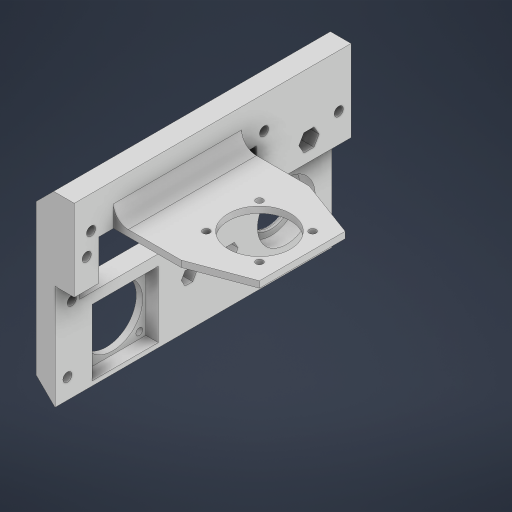
# Autodesk Inventor part: Head_Backplate
Saved by Autodesk Inventor 2024 (Build 280153000, 153)
## iProperties
Created: 2025-09-25
Part Number: Head_Backplate
Material: Generic
Document SubType Name: Modeling
Designer: kevin
Density: 1 g/cm^3
Appearance: Default
Author: kevin
Autodesk Inventor part; units mm, degrees
ref_plane "YZ Plane" through (0, 0, 0) normal (1, 0, 0) x (0, 1, 0)
ref_plane "XZ Plane" through (0, 0, 0) normal (0, 1, 0) x (-1, 0, 0)
sketch "Sketch1" plane through (0, 0, 0) normal (0, 0, 1) x (1, 0, 0)
  line L0 (-40.6109, 70.6994) -> (-33.5378, 59.7448) projected
  line L1 (-33.5378, 59.7448) -> (-15.7647, 71.2203) projected
  line L2 (-15.7647, 71.2203) -> (-15.7647, 87.8486) projected
  line L3 (-15.7647, 87.8486) -> (35.7434, 87.8486) projected
  line L4 (35.7434, 87.8486) -> (-58.3243, 27.112) projected
  line L5 (-58.3243, 27.112) -> (-58.3243, 43.7409) projected
  line L6 (-58.3243, 43.7409) -> (-49.3014, 49.5667) projected
  line L7 (-49.3014, 49.5667) -> (-49.3014, 70.6994) projected
  line L8 (-49.3014, 70.6994) -> (-40.6109, 70.6994) projected
  line L9 (-58.7063, -1.0514) -> (-69.3743, 9.6166) projected
  line L10 (-18.5178, -1.0514) -> (-58.7063, -1.0514) projected
  arc A0 (-21.8066, 1.9486) -> (-18.5178, -1.0514) centre (0, 22.5514) ccw projected
  line L11 (-18.2147, 1.9486) -> (-21.8066, 1.9486) projected
  arc A1 (-18.2147, 1.9486) -> (21.128, 4.9486) centre (0, 22.5514) ccw projected
  line L12 (103.9182, 4.9486) -> (21.128, 4.9486) projected
  line L13 (113.8557, 14.8861) -> (103.9182, 4.9486) projected
  line L14 (113.8557, 93.0111) -> (113.8557, 14.8861) projected
  line L15 (103.9182, 102.9486) -> (113.8557, 93.0111) projected
  line L16 (-46.9118, 102.9486) -> (103.9182, 102.9486) projected
  line L17 (-69.3743, 80.4861) -> (-46.9118, 102.9486) projected
  line L18 (-69.3743, 9.6166) -> (-69.3743, 80.4861) projected
  line L19 (3.2088, 98.8486) -> (52.78, 98.8486) projected
  line L20 (52.78, 98.8486) -> (46.5848, 94.8486) projected
  line L21 (46.5848, 94.8486) -> (5.2088, 94.8486) projected
  line L22 (3.2088, 96.8486) -> (5.2088, 94.8486) projected
  line L23 (3.2088, 96.8486) -> (3.2088, 98.8486) projected
  circle A2 centre (63.0077, 89.467) radius 2.1 projected
  line L24 (67.5987, 76.762) -> (76.5778, 67.7829) projected
  line L25 (76.5778, 67.7829) -> (76.5778, 21.4796) projected
  line L26 (76.5778, 21.4796) -> (68.2692, 13.171) projected
  line L27 (68.2692, 13.171) -> (19.2393, 13.171) projected
  line L28 (19.2393, 13.171) -> (11.6235, 20.7868) projected
  line L29 (11.6235, 20.7868) -> (67.5987, 76.762) projected
  line L30 (-58.0243, 1.9486) -> (-58.0243, 25.3146) projected
  line L31 (-58.0243, -1.0514) -> (-58.0243, 1.9486) projected
  arc A3 (-56.6516, 27.8349) -> (-58.0243, 25.3146) centre (-55.0243, 25.3146) ccw projected
  line L32 (-67.3743, 79.6577) -> (-46.0834, 100.9486)
  line L33 (-46.0834, 100.9486) -> (103.0898, 100.9486)
  line L34 (103.0898, 100.9486) -> (111.8557, 92.1827)
  line L35 (111.8557, 92.1827) -> (111.8557, 15.7145)
  line L36 (111.8557, 15.7145) -> (103.0898, 6.9486)
  line L37 (103.0898, 6.9486) -> (20.1694, 6.9486)
  arc A4 (-17.441, 3.9486) -> (20.1694, 6.9486) centre (0, 22.5514) ccw
  line L38 (-17.441, 3.9486) -> (-26.0372, 3.9486)
  arc A5 (-26.0372, 3.9486) -> (-23.6076, 0.9486) centre (0, 22.5514) ccw
  line L39 (-23.6076, 0.9486) -> (-57.8779, 0.9486)
  line L40 (-57.8779, 0.9486) -> (-67.3743, 10.445) construction
  line L41 (-67.3743, 10.445) -> (-67.3743, 79.6577)
  line L42 (-15.7647, 87.8486) -> (-59.1834, 87.8486)
  line L43 (-49.5014, 70.8994) -> (-49.5014, 49.6757)
  line L44 (-49.5014, 49.6757) -> (-58.5243, 43.8499)
  line L45 (-58.5243, 43.8499) -> (-58.5243, 26.7448)
  line L46 (-58.5243, 26.7448) -> (36.4218, 88.0486)
  line L47 (36.4218, 88.0486) -> (-15.9647, 88.0486)
  line L48 (-15.9647, 88.0486) -> (-15.9647, 71.3293)
  line L49 (-15.9647, 71.3293) -> (-33.4783, 60.0213)
  line L50 (-33.4783, 60.0213) -> (-40.502, 70.8994)
  line L51 (-40.502, 70.8994) -> (-49.5014, 70.8994)
  line L52 (-49.5014, 70.8994) -> (-49.5014, 87.8486)
  line L53 (-58.5243, 26.7448) -> (-58.5243, 1.595)
  line L54 (-67.3743, 9.3192) -> (-58.5243, 0.5765)
  line L55 (-58.5243, 0.5765) -> (-58.5243, 1.595)
  line L56 (-67.3743, 9.3192) -> (-67.3743, 10.445)
  line L57 (-58.5243, 43.8499) -> (-58.5243, 49.6757)
  line L58 (-58.5243, 49.6757) -> (-49.5014, 49.6757)
  point P0 (0, 0)
  dimension "d0" = 2
  dimension "d1" = 0.2
  constraints: 54 end point, 4 point on circle, 3 point on line, 2 centre point, 2 parallel, 2 perpendicular, 1 horizontal, 1 vertical, 19 other
  measures "d0" distance between parallel lines of L18 L41
  measures "d1" distance between parallel lines of L7 L43
ref_plane "Work Plane1" through (-78.2358, -10.3435, 129.6) normal (0, 0, -1) x (0, 1, 0)
extrude "Extrusion1" add sketch "Sketch1" along normal up to surface (129.6 mm away) contours L32 L42 L52 L43 L58 L57 L45 L53 L55 L54 L56 L41
sketch "Sketch2" plane through (-67.3743, 9.3192, 0) normal (-1, 0, 0) x (0, 0, 1)
  circle A0 centre (5.8, 0.6294) radius 2.1 projected
  circle A1 centre (123.8, 0.6294) radius 2.1 projected
  circle A2 centre (123.8, 53.9014) radius 2.1 projected
  circle A3 centre (5.8, 53.9014) radius 2.1 projected
  point P0 (0, -9.3192)
extrude "Extrusion2" cut sketch "Sketch2" against normal blind 25.4
sketch "Sketch4" plane through (-67.3743, 9.3192, 0) normal (-1, 0, 0) x (0, 0, 1)
  arc A0 (125.8035, 0) -> (121.7965, 0) centre (123.8, 0.6294) ccw projected
  line L0 (125.8035, 0) -> (129.6, 0) projected
  line L1 (129.6, 70.3385) -> (129.6, 0) projected
  line L2 (0, 70.3385) -> (129.6, 70.3385) projected
  line L3 (0, 70.3385) -> (0, 0) projected
  line L4 (0, 0) -> (3.7965, 0) projected
  arc A1 (7.8035, 0) -> (3.7965, 0) centre (5.8, 0.6294) ccw projected
  line L5 (7.8035, 0) -> (121.7965, 0) projected
  circle A2 centre (5.8, 53.9014) radius 2.1 projected
  circle A3 centre (123.8, 53.9014) radius 2.1 projected
  circle A4 centre (21.3214, 16.6972) radius 13.5
  point P0 (0, -9.3192)
  dimension "d10" = 27
  constraints: 1 centre point
  measures "d10" diameter of A4
extrude "Extrusion4" cut sketch "Sketch4" against normal up to surface (17.8729 mm away) contours A4
sketch "Sketch5" plane through (-67.3743, 9.3192, 0) normal (-1, 0, 0) x (0, 0, 1)
  circle A0 centre (21.3214, 16.6972) radius 13.5 projected
  circle A1 centre (21.3214, 16.6972) radius 10.325
  point P0 (0, -9.3192)
  dimension "d13" = 20.65
  constraints: 1 centre point, 1 coincident
  measures "d13" diameter of A1
extrude "Extrusion5" add sketch "Sketch5" against normal blind 1.7
fillet "Fillet1" radius 0.6 2 edges at (-67.3743, 26.0164, 10.9964) (-65.6743, 26.0164, 10.9964)
sketch "Sketch7" plane through (-67.3743, 9.3192, 0) normal (-1, 0, 0) x (0, 0, 1)
  circle A0 centre (123.8, 53.9014) radius 2.1 projected
  circle A1 centre (5.8, 53.9014) radius 2.1 projected
  arc A2 (125.8035, 0) -> (121.7965, 0) centre (123.8, 0.6294) ccw projected
  line L0 (125.8035, 0) -> (129.6, 0) projected
  line L1 (129.6, 70.3385) -> (129.6, 0) projected
  line L2 (0, 70.3385) -> (129.6, 70.3385) projected
  line L3 (0, 70.3385) -> (0, 0) projected
  line L4 (0, 0) -> (3.7965, 0) projected
  arc A3 (7.8035, 0) -> (3.7965, 0) centre (5.8, 0.6294) ccw projected
  line L5 (7.8035, 0) -> (121.7965, 0) projected
  circle A4 centre (21.3214, 16.6972) radius 10.925 projected
  circle A5 centre (5.8, 53.9014) radius 3.75
  circle A6 centre (5.8, 0.6294) radius 3.75
  circle A7 centre (123.8, 0.6294) radius 3.75
  circle A8 centre (123.8, 53.9014) radius 3.75
  circle A9 centre (5.8, 0.6294) radius 2.1 projected
  line L6 (2.8, -0.8456) -> (126.8, -0.8456) construction
  circle A10 centre (123.8, 0.6294) radius 2.1 projected
  point P0 (0, -9.3192)
  point P1 (120.1032, 0)
  point P2 (127.4968, 0)
  point P3 (2.1032, 0)
  point P4 (9.4968, 0)
  dimension "d19" = 7.5
  dimension "d20" = 7.5
  dimension "d21" = 7.5
  dimension "d22" = 7.5
  constraints: 4 centre point, 4 coincident
  measures "d19" diameter of A5
  measures "d20" diameter of A6
  measures "d21" diameter of A7
  measures "d22" diameter of A8
extrude "Extrusion7" add sketch "Sketch7" against normal up to surface contours L0 A7 L5 A10 | A6 L4 A9 L5 surface through (-67.3743, 9.3192, 0) normal (-0.7027793, -0.7114079, 0)
sketch "Sketch9" plane through (-67.3743, 9.3192, 0) normal (-1, 0, 0) x (0, 0, 1)
  circle A0 centre (123.8, 53.9014) radius 3.75 projected
  circle A1 centre (5.8, 53.9014) radius 2.1 projected
  circle A2 centre (5.8, 53.9014) radius 3.75
  point P0 (0, -9.3192)
  dimension "d40" = 7.5
  dimension "d41" = 7.5
  constraints: 1 centre point, 1 coincident
  measures "d40" diameter of A2
  measures "d41" diameter of A0
extrude "Extrusion9" cut sketch "Sketch9" against normal blind 4
sketch "Sketch10" plane through (-67.3743, 9.3192, 0) normal (-1, 0, 0) x (0, 0, 1)
  line L0 (50.2647, 59.1822) -> (50.2647, 34.7978) projected
  arc A0 (54.9397, 63.8572) -> (50.2647, 59.1822) centre (54.9397, 59.1822) ccw projected
  line L1 (107.5897, 63.8572) -> (54.9397, 63.8572) projected
  arc A1 (112.2647, 59.1822) -> (107.5897, 63.8572) centre (107.5897, 59.1822) ccw projected
  line L2 (112.2647, 34.7978) -> (112.2647, 59.1822) projected
  arc A2 (107.5897, 30.1228) -> (112.2647, 34.7978) centre (107.5897, 34.7978) ccw projected
  line L3 (54.9397, 30.1228) -> (107.5897, 30.1228) projected
  arc A3 (50.2647, 34.7978) -> (54.9397, 30.1228) centre (54.9397, 34.7978) ccw projected
  circle A4 centre (40.7647, 30.6228) radius 2.1 projected
  circle A5 centre (121.7647, 30.6228) radius 2.1 projected
  circle A6 centre (121.7647, 63.3572) radius 2.1 projected
  circle A7 centre (40.7647, 63.3572) radius 2.1 projected
  line L4 (37.7647, 29.6228) -> (37.7647, 64.3572) projected
  arc A8 (37.7647, 29.6228) -> (39.7647, 27.6228) centre (39.7647, 29.6228) ccw projected
  line L5 (122.7647, 27.6228) -> (39.7647, 27.6228) projected
  arc A9 (122.7647, 27.6228) -> (124.7647, 29.6228) centre (122.7647, 29.6228) ccw projected
  line L6 (124.7647, 64.3572) -> (124.7647, 29.6228) projected
  arc A10 (124.7647, 64.3572) -> (122.7647, 66.3572) centre (122.7647, 64.3572) ccw projected
  line L7 (39.7647, 66.3572) -> (122.7647, 66.3572) projected
  arc A11 (39.7647, 66.3572) -> (37.7647, 64.3572) centre (39.7647, 64.3572) ccw projected
  line L8 (45.4408, 38.9059) -> (45.5414, 50.3571) projected
  line L9 (56.2647, 31.6228) -> (106.2647, 31.6228) projected
  line L10 (116.8647, 50.3572) -> (116.8647, 32.6228) projected
  line L11 (116.8647, 34.6228) -> (116.8647, 32.6228) projected
  line L12 (44.3687, 59.1822) -> (118.1607, 59.1822)
  line L13 (118.1607, 59.1822) -> (118.1607, 29.3503)
  line L14 (118.1607, 29.3503) -> (44.3687, 29.3503)
  line L15 (44.3687, 29.3503) -> (44.3687, 59.1822)
  point P0 (0, -9.3192)
  dimension "d33" = 6.604
  dimension "d34" = 6.604
  constraints: 8 end point, 2 parallel, 1 horizontal, 1 perpendicular
  measures "d33" distance between parallel lines of L4 L15
  measures "d34" distance between parallel lines of L6 L13
extrude "Extrusion10" cut sketch "Sketch10" against normal blind 21.4625 contours L12 L2 A2 L3 A3 L0 | L0 A3 L3 A2 L2 L12 L13 L14 L15 | A4 | A5 | A6 | A7
sketch "Sketch11" plane through (-67.3743, 9.3192, 0) normal (-1, 0, 0) x (0, 0, 1)
  circle A0 centre (40.7647, 63.3572) radius 2.1 projected
  circle A1 centre (121.7647, 63.3572) radius 2.1 projected
  circle A2 centre (40.7647, 30.6228) radius 2.1 projected
  circle A3 centre (121.7647, 30.6228) radius 2.1 projected
  line L0 (118.1607, 29.3503) -> (44.3687, 29.3503) projected
  line L1 (44.3687, 29.3503) -> (44.3687, 59.1822) projected
  line L2 (44.3687, 59.1822) -> (118.1607, 59.1822) projected
  line L3 (118.1607, 59.1822) -> (118.1607, 29.3503) projected
  circle A4 centre (123.8, 53.9014) radius 3.75 projected
  line L4 (127.4968, 0) -> (129.6, 0) projected
  line L5 (129.6, 70.3385) -> (129.6, 0) projected
  line L6 (0, 70.3385) -> (129.6, 70.3385) projected
  line L7 (0, 70.3385) -> (0, 0) projected
  line L8 (0, 0) -> (2.1032, 0) projected
  arc A5 (2.1032, 0) -> (9.4968, 0) centre (5.8, 0.6294) ccw projected
  line L9 (9.4968, 0) -> (120.1032, 0) projected
  arc A6 (120.1032, 0) -> (127.4968, 0) centre (123.8, 0.6294) ccw projected
  circle A7 centre (5.8, 0.6294) radius 2.1 projected
  circle A8 centre (123.8, 0.6294) radius 2.1 projected
  circle A9 centre (21.3214, 16.6972) radius 10.925 projected
  line L10 (11.8, 40.2475) -> (11.8, 61.3802) projected
  line L11 (24.485, 49.283) -> (22.1179, 45.183)
  line L12 (22.1179, 45.183) -> (17.3836, 45.183)
  line L13 (17.3836, 45.183) -> (15.0164, 49.283)
  line L14 (15.0164, 49.283) -> (17.3836, 53.383)
  line L15 (17.3836, 53.383) -> (22.1179, 53.383)
  line L16 (22.1179, 53.383) -> (24.485, 49.283)
  point P0 (0, -9.3192)
  point P1 (19.7507, 49.283)
  dimension "d37" = 8.2
  constraints: 12 end point, 1 parallel, 13 other
  measures "d37" distance between parallel lines of L12 L15
extrude "Extrusion11" cut sketch "Sketch11" against normal blind 21.4625 contours L11 L12 L13 L14 L15 L16
sketch "Sketch12" plane through (-67.3743, 9.3192, 0) normal (-1, 0, 0) x (0, 0, 1)
  line L0 (15.0164, 49.283) -> (17.3836, 53.383) projected
  line L1 (17.3836, 53.383) -> (22.1179, 53.383) projected
  line L2 (22.1179, 53.383) -> (24.485, 49.283) projected
  line L3 (24.485, 49.283) -> (22.1179, 45.183) projected
  line L4 (22.1179, 45.183) -> (17.3836, 45.183) projected
  line L5 (17.3836, 45.183) -> (15.0164, 49.283) projected
  circle A0 centre (40.7647, 63.3572) radius 2.1 projected
  circle A1 centre (121.7647, 63.3572) radius 2.1 projected
  circle A2 centre (40.7647, 30.6228) radius 2.1 projected
  circle A3 centre (121.7647, 30.6228) radius 2.1 projected
  line L6 (118.1607, 29.3503) -> (44.3687, 29.3503) projected
  line L7 (44.3687, 29.3503) -> (44.3687, 59.1822) projected
  line L8 (44.3687, 59.1822) -> (118.1607, 59.1822) projected
  line L9 (118.1607, 59.1822) -> (118.1607, 29.3503) projected
  circle A4 centre (123.8, 53.9014) radius 3.75 projected
  circle A5 centre (5.8, 53.9014) radius 3.75 projected
  line L10 (127.4968, 0) -> (129.6, 0) projected
  line L11 (129.6, 70.3385) -> (129.6, 0) projected
  line L12 (0, 70.3385) -> (129.6, 70.3385) projected
  line L13 (0, 70.3385) -> (0, 0) projected
  line L14 (0, 0) -> (2.1032, 0) projected
  arc A6 (2.1032, 0) -> (9.4968, 0) centre (5.8, 0.6294) ccw projected
  line L15 (9.4968, 0) -> (120.1032, 0) construction
  arc A7 (120.1032, 0) -> (127.4968, 0) centre (123.8, 0.6294) ccw projected
  circle A8 centre (5.8, 0.6294) radius 2.1 projected
  circle A9 centre (123.8, 0.6294) radius 2.1 projected
  circle A10 centre (21.3214, 16.6972) radius 10.925 projected
  arc A11 (120.1032, 0) -> (127.4968, 0) centre (123.8, 0.6294) ccw projected
  line L16 (9.4968, 0) -> (120.1032, 0) projected
  arc A12 (2.1032, 0) -> (9.4968, 0) centre (5.8, 0.6294) ccw projected
  line L17 (0, 0) -> (2.1032, 0) projected
  line L18 (0, 0) -> (0, -8.7427) projected
  line L19 (0, -8.7427) -> (129.6, -8.7427) projected
  line L20 (129.6, 0) -> (129.6, -8.7427) projected
  line L21 (127.4968, 0) -> (129.6, 0) projected
  line L22 (81.7345, 23.8516) -> (111.7345, 23.8516)
  line L23 (111.7345, 23.8516) -> (111.7345, -6.1484)
  line L24 (111.7345, -6.1484) -> (81.7345, -6.1484)
  line L25 (81.7345, -6.1484) -> (81.7345, 23.8516)
  circle A13 centre (84.2845, 21.3016) radius 1.6
  line L26 (96.7345, 23.8516) -> (96.7345, -6.1484) construction
  line L27 (81.7345, 8.8516) -> (111.7345, 8.8516) construction
  circle A14 centre (109.1845, 21.3016) radius 1.6
  circle A15 centre (84.2845, -3.5984) radius 1.6
  circle A16 centre (109.1845, -3.5984) radius 1.6
  line L28 (79.7345, -8.1484) -> (113.7345, -8.1484)
  line L29 (113.7345, -8.1484) -> (113.7345, 25.8516)
  line L30 (113.7345, 25.8516) -> (79.7345, 25.8516)
  line L31 (79.7345, 25.8516) -> (79.7345, -8.1484)
  circle A17 centre (96.7345, 8.8516) radius 14
  line L32 (81.2345, 24.3516) -> (112.2345, 24.3516)
  line L33 (112.2345, 24.3516) -> (112.2345, -6.6484)
  line L34 (112.2345, -6.6484) -> (81.2345, -6.6484)
  line L35 (81.2345, -6.6484) -> (81.2345, 24.3516)
  point P0 (0, -9.3192)
  point P1 (113.7345, 0)
  point P2 (112.2345, 0)
  point P3 (81.2345, 0)
  point P4 (79.7345, 0)
  dimension "d42" = 30
  dimension "d43" = 30
  dimension "d44" = 3.2
  dimension "d45" = 2.55
  dimension "d46" = 2.55
  dimension "d47" = 2
  dimension "d48" = 28
  dimension "d49" = 0.5
  constraints: 28 end point, 6 parallel, 5 centre point, 5 midpoint, 3 perpendicular, 3 symmetric about line, 1 horizontal, 9 other
  measures "d42" distance of L23.end L24.end
  measures "d43" distance of L22.end L23.end
  measures "d44" diameter of A13
  measures "d45" distance from line of L22 A13.centre
  measures "d46" distance from line of L25 A13.centre
  measures "d47" distance between parallel lines of L24 L28
  measures "d48" diameter of A17
  measures "d49" distance between parallel lines of L25 L35
extrude "Extrusion12" cut sketch "Sketch12" against normal blind 13.525 contours L33 L34 L35 L16 L25 L24 L23 | L16 L23 L22 L25 L35 L32 L33 | L23 L24 L25 L16 A17 | L16 A17 L25 L22 L23 | A17 L16 | L16 A17 | A13 | A14 | A15 | A16
extrude "Extrusion13" add sketch "Sketch12" against normal up to surface contours L29 L28 L31 L16 L35 L34 L33 surface through (-67.3743, 9.3192, 0) normal (-0.7027793, -0.7114079, 0)
extrude "Extrusion14" add sketch "Sketch12" against normal blind 3 contours L33 L34 L35 L16 L25 L24 L23 | L16 L23 L22 L25 L35 L32 L33 | L23 L24 L25 L16 A17 | L16 A17 L25 L22 L23
sketch "Sketch13" plane through (-67.3743, 9.3192, 0) normal (-1, 0, 0) x (0, 0, 1)
  line L0 (39.8496, 4.3144) -> (74.556, 4.3144)
  line L1 (74.556, 4.3144) -> (74.556, 21.9591)
  line L2 (74.556, 21.9591) -> (39.8496, 21.9591)
  line L3 (39.8496, 21.9591) -> (39.8496, 4.3144)
  line L4 (39.8496, 4.3144) -> (74.556, 21.9591) construction
  line L5 (74.556, 4.3144) -> (39.8496, 21.9591) construction
  line L6 (43.89, 13.1368) -> (45.6798, 16.2368)
  line L7 (45.6798, 16.2368) -> (49.2594, 16.2368)
  line L8 (49.2594, 16.2368) -> (51.0492, 13.1368)
  line L9 (51.0492, 13.1368) -> (49.2594, 10.0368)
  line L10 (49.2594, 10.0368) -> (45.6798, 10.0368)
  line L11 (45.6798, 10.0368) -> (43.89, 13.1368)
  line L12 (63.3565, 13.1368) -> (65.1462, 16.2368)
  line L13 (65.1462, 16.2368) -> (68.7258, 16.2368)
  line L14 (68.7258, 16.2368) -> (70.5156, 13.1368)
  line L15 (70.5156, 13.1368) -> (68.7258, 10.0368)
  line L16 (68.7258, 10.0368) -> (65.1462, 10.0368)
  line L17 (65.1462, 10.0368) -> (63.3565, 13.1368)
  line L18 (118.1607, 29.3503) -> (44.3687, 29.3503) projected
  line L19 (39.8496, 13.1368) -> (74.556, 13.1368) construction
  point P0 (0, -9.3192)
  point P1 (57.2028, 13.1368)
  point P2 (47.4696, 13.1368)
  point P3 (66.936, 13.1368)
  dimension "d56" = 6.2
  dimension "d57" = 6.2
  dimension "d58" = 7.62
  dimension "d59" = 7.62
  constraints: 38 end point, 4 midpoint, 4 parallel, 1 horizontal, 1 perpendicular, 26 other
  measures "d56" distance between parallel lines of L10 L7
  measures "d57" distance between parallel lines of L16 L13
  measures "d58" distance from line of L1 point (66.936, 13.137)
  measures "d59" distance from line of L3 point (47.47, 13.137)
extrude "Extrusion15" cut sketch "Sketch13" against normal blind 12.525 contours L6 L7 L8 L9 L10 L11 | L12 L13 L14 L15 L16 L17
sketch "Sketch14" plane through (-49.5014, 49.6757, 0) normal (1, 0, 0) x (0, 0, -1)
  line L0 (-17.3836, 13.0266) -> (-15.0164, 8.9266) projected
  line L1 (-15.0164, 8.9266) -> (-17.3836, 4.8266) projected
  line L2 (-17.3836, 4.8266) -> (-22.1179, 4.8266) projected
  line L3 (-22.1179, 4.8266) -> (-24.485, 8.9266) projected
  line L4 (-24.485, 8.9266) -> (-22.1179, 13.0266) projected
  line L5 (-22.1179, 13.0266) -> (-17.3836, 13.0266) projected
  line L6 (-44.3687, 18.8257) -> (-44.3687, 0) projected
  line L7 (0, 0) -> (-44.3687, 0) projected
  line L8 (0, 0) -> (0, 38.1729) projected
  line L9 (0, 38.1729) -> (-129.6, 38.1729) projected
  line L10 (-129.6, 0) -> (-129.6, 38.1729) projected
  line L11 (-118.1607, 0) -> (-129.6, 0) projected
  line L12 (-118.1607, 0) -> (-118.1607, 18.8257) projected
  line L13 (-118.1607, 18.8257) -> (-44.3687, 18.8257) projected
  circle A0 centre (-40.7647, 23.0007) radius 2.1 projected
  circle A1 centre (-121.7647, 23.0007) radius 2.1 projected
  circle A2 centre (-123.8, 13.5449) radius 2.1 projected
  circle A3 centre (-5.8, 13.5449) radius 2.1 projected
  line L14 (-81.2647, 18.8257) -> (-81.2647, -105.8189) construction
  line L15 (-111.2647, 18.8257) -> (-51.2647, 18.8257)
  line L16 (-51.2647, 18.8257) -> (-51.2647, 21.8257)
  line L17 (-51.2647, 21.8257) -> (-111.2647, 21.8257)
  line L18 (-111.2647, 21.8257) -> (-111.2647, 18.8257)
  line L19 (-81.2647, 21.8257) -> (-81.2647, 18.8257) construction
  line L20 (-118.1607, 18.8257) -> (-44.3687, 18.8257) construction
  point P0 (0, -49.6757)
  dimension "d62" = 3
  dimension "d69" = 60
  constraints: 12 end point, 4 midpoint, 2 parallel, 2 point on line, 1 horizontal, 1 perpendicular, 1 vertical
  measures "d62" distance of L16.end L15.end
  measures "d69" distance of L16.end L17.end
extrude "Extrusion16" add sketch "Sketch14" along normal blind 63.325 contours L13 L18 L17 L16
sketch "Sketch15" plane through (-49.5014, 71.5014, 111.2647) normal (0, 1, 0) x (1, 0, 0)
  line L0 (0, 0) -> (0, 60) projected
  line L1 (0, 0) -> (63.325, 0) projected
  line L2 (63.325, 60) -> (63.325, 0) projected
  line L3 (0, 60) -> (63.325, 60) projected
  line L4 (45.4626, 33.0804) -> (30.7499, 33.0804) construction
  line L5 (30.7499, 33.0804) -> (30.7499, 18.0559) construction
  line L6 (30.7499, 18.0559) -> (45.9614, 18.0559) construction
  line L7 (45.9614, 18.0559) -> (45.9614, 32.4881) construction
  line L8 (45.9614, 32.4881) -> (45.4626, 33.0804) construction
  line L9 (38.3556, 0) -> (38.3556, 60) construction
  line L10 (53.3556, 15) -> (23.3556, 15)
  line L11 (23.3556, 15) -> (23.3556, 45)
  line L12 (23.3556, 45) -> (53.3556, 45)
  line L13 (53.3556, 45) -> (53.3556, 15)
  line L14 (53.3556, 15) -> (23.3556, 45) construction
  line L15 (23.3556, 15) -> (53.3556, 45) construction
  circle A0 centre (50.8056, 42.45) radius 1.6
  circle A1 centre (25.9056, 42.45) radius 1.6
  line L16 (38.3556, 30) -> (43.1871, 30) construction
  circle A2 centre (50.8056, 17.55) radius 1.6
  circle A3 centre (25.9056, 17.55) radius 1.6
  circle A4 centre (38.3556, 30) radius 14.5
  line L17 (31.6625, 60) -> (58.4228, 50.0671)
  line L18 (58.4228, 50.0671) -> (58.4228, 30)
  line L19 (31.6625, 0) -> (58.4228, 9.9329)
  line L20 (58.4228, 9.9329) -> (58.4228, 30)
  point P0 (49.5014, 111.2647)
  point P1 (31.6625, 0)
  dimension "d67" = 30
  dimension "d68" = 30
  dimension "d70" = 3.2
  dimension "d71" = 2.55
  dimension "d72" = 2.55
  dimension "d73" = 29
  constraints: 24 end point, 5 centre point, 5 symmetric about line, 4 midpoint, 2 horizontal, 2 parallel, 2 perpendicular, 2 point on line, 1 coincident, 1 vertical, 3 other
  measures "d67" distance of L11.end L12.end
  measures "d68" distance of L10.end L11.end
  measures "d70" diameter of A0
  measures "d71" distance from line of L13 A0.centre
  measures "d72" distance from line of L12 A0.centre
  measures "d73" diameter of A4
extrude "Extrusion17" cut sketch "Sketch15" against normal blind 63.325 contours L19 L20 L18 L17 L3 L2 L1 | A0 | A1 | A2 | A3 | A4
fillet "Fillet2" radius 6.95 1 edges at (-49.5014, 71.5014, 81.2647)
chamfer "Chamfer1" distance 1 angle 45 1 edges at (-67.3743, 1.1708, 96.7345)
equation "\"d40\" = d41"
equation "\"d46\" = d45"
equation "\"d59\" = d58"
equation "\"d72\" = d71"
body "Solid1"
